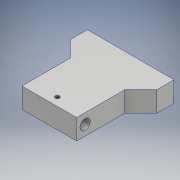
# Autodesk Inventor part: suporte_guia_central
Saved by Autodesk Inventor 2018 (Build 220112000, 112)
## iProperties
Created: 2018-05-16
Part Number: suporte_guia_central
Material: Alumínio 6061
Document SubType Name: Modeling
Designer: Usuario
Density: 2.7 g/cm^3
Appearance: Alumínio - Plano
Mass: 482.085 g
Surface Area: 275.155 cm^2
Volume: 178.55 cm^3
Author: Usuario
Autodesk Inventor part; units mm, degrees
ref_plane "YZ Plane" through (0, 0, 0) normal (1, 0, 0) x (0, 1, 0)
ref_plane "XZ Plane" through (0, 0, 0) normal (0, 1, 0) x (-1, 0, 0)
ref_plane "XY Plane" through (0, 0, 0) normal (0, 0, 1) x (1, 0, 0)
sketch "Esboço1" plane through (0, 0, 0) normal (0, 0, 1) x (1, 0, 0)
  line L0 (0, 36.3068) -> (0, -8.6932) construction
  circle A0 centre (0, -8.6932) radius 68 construction
  line L1 (0, 36.3068) -> (50.9804, 36.3068)
  line L2 (50.9804, 36.3068) -> (50.9804, 16.3068)
  line L3 (50.9804, 16.3068) -> (32.1355, -2.5381)
  line L4 (32.1355, -2.5381) -> (32.1355, -59.5381)
  line L5 (32.1355, -59.5381) -> (0, -59.5381)
  line L6 (0, -76.6932) -> (0, 59.3068) construction
  line L7 (0, 36.3068) -> (-50.9804, 36.3068)
  line L8 (-50.9804, 36.3068) -> (-50.9804, 16.3068)
  line L9 (-50.9804, 16.3068) -> (-32.1355, -2.5381)
  line L10 (-32.1355, -2.5381) -> (-32.1355, -59.5381)
  line L11 (-32.1355, -59.5381) -> (0, -59.5381)
  point P0 (0, 0)
  dimension "d1" = 45
  dimension "d2" = 136
  dimension "d3" = 20
  dimension "d4" = 135
  dimension "d5" = 57
  dimension "d7" = 50.9804
  dimension "d41" = 32.1355
  constraints: 24 end point, 4 symmetric about line, 3 perpendicular, 3 point on circle, 1 centre point, 1 coincident, 1 collinear, 1 vertical, 1 other
  measures "d1" distance of L0.start L0.end
  measures "d2" diameter of A0
  measures "d3" distance of L1.end L2.end
  measures "d4" angle of L2 L3
  measures "d5" distance of L3.end L4.end
  measures "d7" distance of L0.start L1.end
  measures "d41" distance of L4.end L5.end
extrude "Extrusão1" add sketch "Esboço1" along normal mid plane 24
sketch "Esboço2" plane through (-32.1355, -59.5381, 12) normal (-1, 0, 0) x (0, 0, 1)
  line L0 (0, 0) -> (-24, 0) construction
  line L1 (-12, 0) -> (-12, 10) construction
  circle A0 centre (-12, 10) radius 6.075
  point P0 (-12, 59.5381)
  dimension "d10" = 10
  dimension "d11" = 12.15
  constraints: 2 end point, 1 centre point, 1 coincident, 1 midpoint, 1 vertical
  measures "d10" distance of L1.start L1.end
  measures "d11" diameter of A0
hole "Furo1" at (-32.1355, -49.5381, 0) direction (1, 0, 0) diameter 12.15 end through all
sketch "Esboço3" plane through (0, 0, 12) normal (0, 0, 1) x (1, 0, 0)
  line L0 (0, 0) -> (0, -50) construction
  dimension "d42" = 50
  constraints: 2 end point, 1 vertical
  measures "d42" distance of L0.start L0.end
hole "Furo2" at (0, -50, 12) direction (0, 0, -1) diameter 4.917 depth 10 tip angle 118 thread size "M6x1" class "6H" standard "ANSI Metric M Profile"
